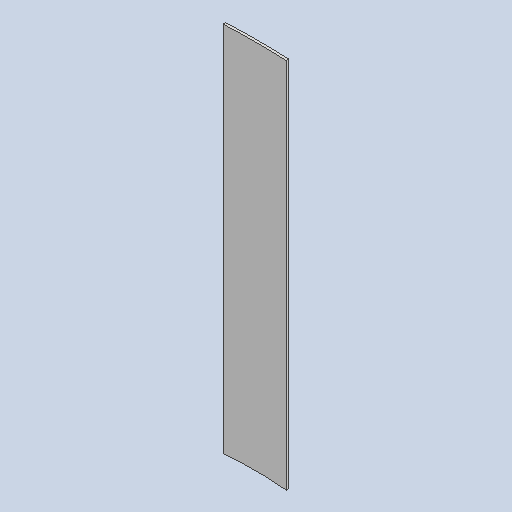
# Autodesk Inventor part: DMF 01 12 Барабан усилитель v2.1
Saved by Autodesk Inventor 2025 (Build 290162010, 162A)
## iProperties
Created: 2024-04-30
Part Number: DMF 01 12 Барабан усилитель v2.1
Material: Generic
Document SubType Name: Sheet Metal
Designer: admin
Density: 1 g/cm^3
Sheet Metal Rule: Default
Appearance: Default
Sheet Metal Width: 0,000 mm
Sheet Metal Length: 0,000 mm
Sheet Metal Area: 0,000 mm^2
Stock Number: Барабан_Сектор_Усилителя
Author: pokla
Autodesk Inventor part; units mm, degrees
ref_plane "YZ Plane" through (0, 0, 0) normal (1, 0, 0) x (0, 1, 0)
ref_plane "XZ Plane" through (0, 0, 0) normal (0, 1, 0) x (-1, 0, 0)
ref_plane "XY Plane" through (0, 0, 0) normal (0, 0, 1) x (1, 0, 0)
sketch "Sketch1" plane through (0, 0, 0) normal (0, 0, 1) x (1, 0, 0)
  circle A0 centre (0, 0) radius 256
  line L0 (-25, 549.4315) -> (25, 549.4315)
  line L1 (25, 549.4315) -> (25, 254.7764)
  line L2 (25, 254.7764) -> (-25, 254.7764)
  line L3 (-25, 254.7764) -> (-25, 549.4315)
  circle A1 centre (0, 0) radius 550
  dimension "d28" = 1100
  dimension "d26" = 512
  dimension "d27" = 50
  measures "d26" diameter of A0
  measures "d27" distance of L1.end L2.end
extrude "Plate1" add sketch "Sketch1" against normal blind 2 contours A0 L3 L0 L1 | L0 A1
equation "\"d28\" = Колесо_диам2_ручья_внутр"
equation "\"d26\" = Колесо_диам3_борт_ступицы + 2 * Thickness"
equation "\"d15\" = Thickness"
equation "\"BendRadius\" = Thickness"
equation "\"BendReliefWidth\" = Thickness"
equation "\"BendReliefDepth\" = 0.5 * Thickness"
equation "\"CornerReliefSize\" = 4 * Thickness"
equation "\"MinimumRemnant\" = 2 * Thickness"
equation "\"TransitionRadius\" = BendRadius"
equation "\"JacobiRadiusSize\" = BendRadius"
equation "\"GapSize\" = Thickness"
equation "\"Колесо_диам2_ручья_внутр\" = 1100"
equation "\"Колесо_диам3_борт_ступицы\" = 508"
equation "\"Thickness\" = 2"
body "Solid1"
